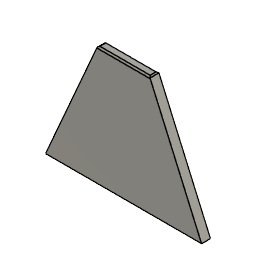
BRC fins (Autodesk Fusion 360 design; units mm, degrees)
part number: 2026-02-28-15-39-29-449
Autodesk Fusion 360 part; units mm, degrees
sketch "Sketch1" plane through (0, 0, 0) normal (0, 1, 0) x (1, 0, 0)
  line L0 (-50, 0) -> (55, 0)
  line L1 (-15, -80) -> (20, -80)
  line L2 (-50, 0) -> (-15, -80)
  line L3 (20, -80) -> (55, 0)
  dimension "d2" = 105
  dimension "d3" = 35
  dimension "d4" = 35
  dimension "d5" = 80
  dimension "d6" = 50
  constraint horizontal L0
  constraint horizontal L1
  constraint horizontal origin L0.start
  measures "d2" distance of L0.start L0.end
  measures "d3" distance of L1.start L1.end
  measures "d4" horizontal distance of L0.start L1.start
  measures "d5" distance of L0 L1
  measures "d6" horizontal distance of origin L0.start
extrude "Extrude1" add sketch "Sketch1" along normal mid plane 6
fillet "Fillet1" radius 1 4 edges at (2.5, -3, 80) (2.5, 3, 80) (-15, 0, 80) (20, 0, 80)
chamfer "Chamfer1" distance 0.5 distance2 1 4 edges at (2.5, -3, 0) (2.5, 3, 0) (-50, 0, 0) (55, 0, 0) measured on face at (-3.4792, -3, 26.3333) measured on face at (-3.4792, 3, 26.3333) measured on face at (-26.9583, 1, 52.6667) measured on face at (31.9583, -1, 52.6667)
